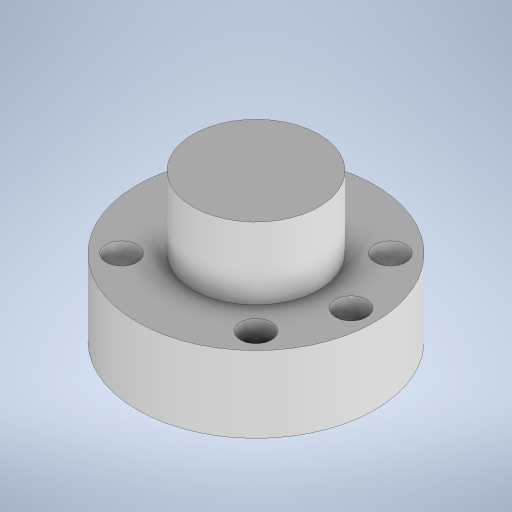
# Autodesk Inventor part: SoporteIRB
Saved by Autodesk Inventor 2023 (Build 270158000, 158)
## iProperties
Created: 2022-08-30
Part Number: SoporteIRB
Material: Generic
Document SubType Name: Modeling
Designer: andre
Density: 1 g/cm^3
Appearance: Default
Author: andre
Autodesk Inventor part; units mm, degrees
ref_plane "YZ Plane" through (0, 0, 0) normal (1, 0, 0) x (0, 1, 0)
ref_plane "XZ Plane" through (0, 0, 0) normal (0, 1, 0) x (-1, 0, 0)
sketch "Sketch1" plane through (0, 0, 0) normal (0, 0, 1) x (1, 0, 0)
  circle A0 centre (0, 0) radius 25
  dimension "d0" = 50
  constraints: 1 centre point, 1 coincident
  measures "d0" diameter of A0
extrude "Extrusion1" add sketch "Sketch1" along normal blind 16
sketch "Sketch2" plane through (0, 0, 16) normal (0, 0, 1) x (1, 0, 0)
  line L0 (0, 0) -> (-14.1421, 14.1421)
  line L1 (0, 0) -> (-17.9491, 0)
  point P0 (-14.1421, -14.1421)
  point P1 (-14.1421, -14.1421)
  point P2 (14.1421, -14.1421)
  point P3 (14.1421, -14.1421)
  point P4 (14.1421, 14.1421)
  point P5 (14.1421, 14.1421)
  point P6 (0, 20)
  dimension "d3" = 45
  dimension "d4" = 20
  dimension "d7" = 360
  dimension "d9" = 20
  constraints: 4 coincident, 4 end point, 1 horizontal, 9 other
  measures "d3" angle of L0 L1
  measures "d4" distance of L0.start L0.end
  measures "d9" distance from line of point (0, 20) L1
hole "Hole1" at (-14.1421, 14.1421, 16) at (-14.1421, -14.1421, 16) at (14.1421, -14.1421, 16) at (14.1421, 14.1421, 16) at (0, 20, 16) direction (0, 0, -1) diameter 6.5 end through all
sketch "Sketch3" plane through (0, 0, 16) normal (0, 0, 1) x (1, 0, 0)
  circle A0 centre (0, 0) radius 13.25
  dimension "d17" = 26.5
  constraints: 1 centre point, 1 coincident
  measures "d17" diameter of A0
extrude "Extrusion2" add sketch "Sketch3" along normal blind 15.1
sketch "Sketch4" plane through (0, 0, 31.1) normal (0, 0, 1) x (1, 0, 0)
  circle A0 centre (0, 0) radius 13.25 projected
  point P0 (13.25, 0)
  constraints: 1 horizontal alignment, 1 other
ref_plane "Work Plane1" through (13.25, 0, 31.1) normal (1, 0, 0) x (0, 1, 0)
body "Solid1"
